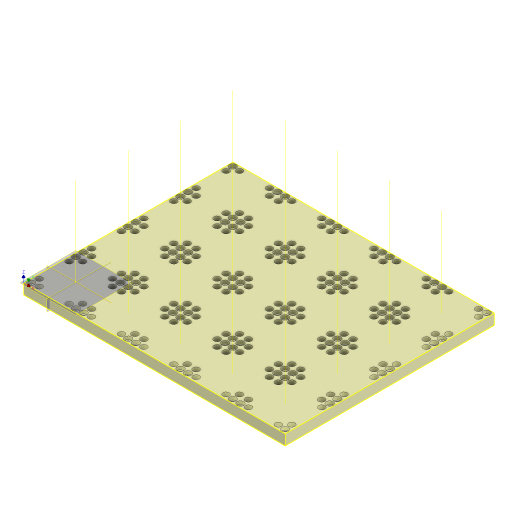
# Autodesk Inventor part: TMP_Plate_Münster
Saved by Autodesk Inventor 2024.1 (Build 281209000, 209)
## iProperties
Created: 2024-08-02
Part Number: TMP_Plate_Münster
Material: Generisch
Document SubType Name: Modeling
Designer: diederichbenedict
Density: 1 g/cm^3
Appearance: Vorgabe
Author: diederichbenedict
Autodesk Inventor part; units mm, degrees
ref_plane "YZ Plane" through (0, 0, 0) normal (1, 0, 0) x (0, 1, 0)
ref_plane "XZ Plane" through (0, 0, 0) normal (0, 1, 0) x (-1, 0, 0)
ref_plane "XY Plane" through (0, 0, 0) normal (0, 0, 1) x (1, 0, 0)
ref_plane "Arbeitsebene1" through (211.7743, 99.4885, -62.2035) normal (0, 0, -1) x (-1, 0, 0)
sketch "Skizze1" plane through (211.7743, 99.4885, -62.2035) normal (0, 0, -1) x (-1, 0, 0)
  circle A0 centre (20.71, 14.3) radius 2.475 projected
  circle A1 centre (14.3, -20.71) radius 2.475 projected
  circle A2 centre (-20.71, -14.3) radius 2.475 projected
  circle A3 centre (-14.3, 20.71) radius 2.475 projected
  circle A4 centre (14.3, 20.71) radius 2.475 projected
  circle A5 centre (-20.71, 14.3) radius 2.475 projected
  circle A6 centre (-14.3, -20.71) radius 2.475 projected
  circle A7 centre (20.71, -14.3) radius 2.475 projected
  line L0 (-17.02, -17.02) -> (-17.02, 17.02) projected
  line L1 (-17.02, 17.02) -> (17.02, 17.02) projected
  line L2 (17.02, 17.02) -> (17.02, -17.02) projected
  line L3 (17.02, -17.02) -> (-17.02, -17.02) projected
  circle A8 centre (-21.25, -21.25) radius 2.75 projected
  circle A9 centre (21.25, 21.25) radius 2.75 projected
  arc A10 (-24.4, -22.9) -> (-22.9, -24.4) centre (-22.9, -22.9) ccw projected
  line L4 (22.9, -24.4) -> (-22.9, -24.4) projected
  arc A11 (22.9, -24.4) -> (24.4, -22.9) centre (22.9, -22.9) ccw projected
  line L5 (24.4, 22.9) -> (24.4, -22.9) projected
  arc A12 (24.4, 22.9) -> (22.9, 24.4) centre (22.9, 22.9) ccw projected
  line L6 (-22.9, 24.4) -> (22.9, 24.4) projected
  arc A13 (-22.9, 24.4) -> (-24.4, 22.9) centre (-22.9, 22.9) ccw projected
  line L7 (-24.4, -22.9) -> (-24.4, 22.9) projected
  line L8 (-25, -25) -> (25, -25)
  line L9 (25, -25) -> (25, 25)
  line L10 (25, 25) -> (-25, 25)
  line L11 (-25, 25) -> (-25, -25)
  line L12 (-25, -25) -> (25, 25) construction
  line L13 (25, -25) -> (-25, 25) construction
  circle A14 centre (21.25, 21.25) radius 1.4
  line L14 (-21.3324, -21.3324) -> (21.3324, -21.3324) construction
  line L15 (21.3324, -21.3324) -> (21.3324, 21.3324) construction
  line L16 (21.3324, 21.3324) -> (-21.3324, 21.3324) construction
  line L17 (-21.3324, 21.3324) -> (-21.3324, -21.3324) construction
  line L18 (-21.3324, -21.3324) -> (21.3324, 21.3324) construction
  line L19 (21.3324, -21.3324) -> (-21.3324, 21.3324) construction
  circle A15 centre (21.3324, -21.3324) radius 1.4
  circle A16 centre (-21.3324, -21.3324) radius 1.4
  circle A17 centre (-21.3324, 21.3324) radius 1.4
  circle A18 centre (20.71, 14.3) radius 3
  circle A19 centre (20.71, -14.3) radius 3
  circle A20 centre (14.3, -20.71) radius 3
  circle A21 centre (-14.3, -20.71) radius 3
  circle A22 centre (-20.71, -14.3) radius 3
  circle A23 centre (-20.71, 14.3) radius 3
  circle A24 centre (-14.3, 20.71) radius 3
  circle A25 centre (14.3, 20.71) radius 3
  point P0 (211.7743, -99.4885)
  point P1 (0, 0)
  dimension "d0" = 50
  dimension "d1" = 50
  dimension "d2" = 2.8
  dimension "d3" = 2.8
  dimension "d4" = 2.8
  dimension "d5" = 2.8
  dimension "d20" = 6
  dimension "d7" = 6
  dimension "d8" = 6
  dimension "d9" = 6
  dimension "d10" = 6
  dimension "d11" = 6
  dimension "d12" = 6
  dimension "d13" = 6
  constraints: 24 end point, 12 centre point, 12 coincident, 4 midpoint, 4 parallel, 2 horizontal, 2 perpendicular, 1 point on line
  measures "d0" distance of L10.end L9.end
  measures "d1" distance of L9.end L8.end
  measures "d2" diameter of A14
  measures "d3" diameter of A15
  measures "d4" diameter of A16
  measures "d5" diameter of A17
  measures "d20" diameter of A18
  measures "d7" diameter of A19
  measures "d8" diameter of A20
  measures "d9" diameter of A21
  measures "d10" diameter of A22
  measures "d11" diameter of A23
  measures "d12" diameter of A24
  measures "d13" diameter of A25
extrude "Extrusion1" add sketch "Skizze1" along normal blind 10 contours L0 L1 L2 L3 | A8 | A9 | L7 A13 L6 A12 L5 A11 L4 A10 | L11 L10 L9 L8
sketch "Skizze2" plane through (211.7743, 99.4885, -62.2035) normal (0, 0, 1) x (1, 0, 0)
  line L0 (-25, -25) -> (-25, 25) projected
  line L1 (25, -25) -> (-25, -25) projected
  line L2 (25, 25) -> (25, -25) projected
  line L3 (-25, 25) -> (25, 25) projected
  circle A0 centre (21.3324, -21.3324) radius 1.4 projected
  circle A1 centre (-21.25, 21.25) radius 1.4 projected
  circle A2 centre (-20.71, 14.3) radius 3 projected
  circle A3 centre (-20.71, -14.3) radius 3 projected
  circle A4 centre (-14.3, -20.71) radius 3 projected
  circle A5 centre (14.3, -20.71) radius 3 projected
  circle A6 centre (20.71, -14.3) radius 3 projected
  circle A7 centre (20.71, 14.3) radius 3 projected
  circle A8 centre (14.3, 20.71) radius 3 projected
  circle A9 centre (-14.3, 20.71) radius 3 projected
  circle A10 centre (21.3324, 21.3324) radius 1.4 projected
  circle A11 centre (-21.3324, -21.3324) radius 1.4 projected
  point P0 (-211.7743, -99.4885)
hole "Bohrung1" at (233.1067, 120.8209, -62.2035) at (233.1067, 78.1561, -62.2035) at (190.442, 78.1561, -62.2035) at (190.5243, 120.7385, -62.2035) direction (0, 0, -1) diameter 3.5 end through all counterbore diameter 6.5 counterbore depth 3
sketch "Skizze3" plane through (211.7743, 99.4885, -72.2035) normal (0, 0, -1) x (-1, 0, 0)
  circle A0 centre (21.25, 21.25) radius 1.75 projected
  circle A1 centre (21.3324, -21.3324) radius 1.75 projected
  circle A2 centre (-21.3324, -21.3324) radius 1.75 projected
  circle A3 centre (-21.3324, 21.3324) radius 1.75 projected
  line L0 (25, -25) -> (25, 25) projected
  line L1 (25, 25) -> (-25, 25) projected
  line L2 (-25, 25) -> (-25, -25) projected
  line L3 (-25, -25) -> (25, -25) projected
  circle A4 centre (20.71, 14.3) radius 3 projected
  circle A5 centre (20.71, -14.3) radius 3 projected
  circle A6 centre (14.3, -20.71) radius 3 projected
  circle A7 centre (-14.3, -20.71) radius 3 projected
  circle A8 centre (-20.71, -14.3) radius 3 projected
  circle A9 centre (-20.71, 14.3) radius 3 projected
  circle A10 centre (-14.3, 20.71) radius 3 projected
  circle A11 centre (14.3, 20.71) radius 3 projected
  line L4 (-22.3198, 16.1722) -> (-19.8935, 16.6303)
  line L5 (-19.8935, 16.6303) -> (-18.2837, 14.758)
  line L6 (-18.2837, 14.758) -> (-19.1002, 12.4278)
  line L7 (-19.1002, 12.4278) -> (-21.5265, 11.9697)
  line L8 (-21.5265, 11.9697) -> (-23.1363, 13.842)
  line L9 (-23.1363, 13.842) -> (-22.3198, 16.1722)
  line L10 (-12.6325, 22.5563) -> (-11.8673, 20.1891)
  line L11 (-11.8673, 20.1891) -> (-13.5347, 18.3428)
  line L12 (-13.5347, 18.3428) -> (-15.9675, 18.8637)
  line L13 (-15.9675, 18.8637) -> (-16.7327, 21.2309)
  line L14 (-16.7327, 21.2309) -> (-15.0653, 23.0772)
  line L15 (-15.0653, 23.0772) -> (-12.6325, 22.5563)
  circle A12 centre (-20.71, 14.3) radius 2.45 construction
  circle A13 centre (-14.3, 20.71) radius 2.45 construction
  point P0 (211.7743, -99.4885)
  dimension "d30" = 4.9
  dimension "d31" = 4.9
  constraints: 24 end point, 4 coincident, 2 centre point, 26 other
  measures "d30" diameter of A12
  measures "d31" diameter of A13
extrude "Extrusion2" add sketch "Skizze3" against normal blind 5 contours A9 | A10
ref_plane "Arbeitsebene2" through (186.7743, 99.4885, -62.2035) normal (0, -1, 0) x (1, 0, 0)
ref_plane "Arbeitsebene3" through (211.7743, 74.4885, -62.2035) normal (-1, 0, 0) x (0, 0, 1)
pattern_circular "Runde Anordnung1" count 4 over 360 about axis through (211.7743, 99.4885, -62.2035) along (0, 0, -1) of "Extrusion2"
pattern_linear "Rechteckige Anordnung2" count 5 spacing 50 along (1, 0, 0) count 4 spacing 50 along (0, 1, 0) of "Extrusion1", "Bohrung1", "Extrusion2", "Runde Anordnung1"
equation "\"d0\" = d1"
